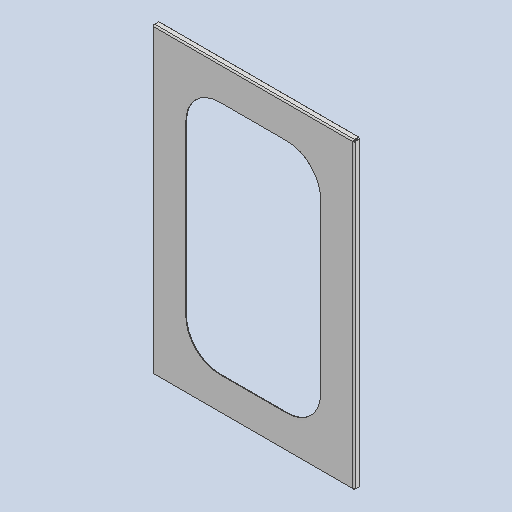
# Autodesk Inventor part: TapaCentral
Saved by Autodesk Inventor 2023 (Build 270158000, 158)
## iProperties
Created: 2022-11-27
Part Number: TapaCentral
Material: Generic
Document SubType Name: Sheet Metal
Designer: David
Density: 1 g/cm^3
Sheet Metal Rule: Default
Appearance: Default
Flat Pattern Width: 138.94 cm
Flat Pattern Length: 93.9405 cm
Flat Pattern Area: 13052.1 cm^2
Sheet Metal Width: 1389,405 mm
Sheet Metal Length: 939,405 mm
Sheet Metal Area: 1305213,601 mm^2
Author: David
Autodesk Inventor part; units mm, degrees
note: some values were not read from the file. Chosen so that the rebuilt part matches the saved one: corner form of "Plate4".
ref_plane "YZ Plane" through (0, 0, 0) normal (1, 0, 0) x (0, 1, 0)
ref_plane "XZ Plane" through (0, 0, 0) normal (0, 1, 0) x (-1, 0, 0)
ref_plane "XY Plane" through (0, 0, 0) normal (0, 0, 1) x (1, 0, 0)
sketch "Sketch1" plane through (0, 0, 0) normal (0, 0, 1) x (1, 0, 0)
  line L0 (-450, -675) -> (450, -675)
  line L1 (450, -675) -> (450, 675)
  line L2 (450, 675) -> (-450, 675)
  line L3 (-450, 675) -> (-450, -675)
  line L4 (-450, -675) -> (450, 675) construction
  line L5 (450, -675) -> (-450, 675) construction
  line L6 (-150, 525) -> (150, 525)
  line L7 (300, 375) -> (300, -375)
  line L8 (150, -525) -> (-150, -525)
  line L9 (-300, -375) -> (-300, 375)
  arc A0 (300, 375) -> (150, 525) centre (150, 375) ccw
  arc A1 (-150, 525) -> (-300, 375) centre (-150, 375) ccw
  arc A2 (-300, -375) -> (-150, -525) centre (-150, -375) ccw
  arc A3 (150, -525) -> (300, -375) centre (150, -375) ccw
  point P0 (0, 0)
  dimension "d0" = 900
  dimension "d1" = 1350
  dimension "d13" = 150
  dimension "d14" = 150
  dimension "d15" = 150
  dimension "d16" = 150
  dimension "d17" = 150
  measures "d0" distance of L2.end L1.end
  measures "d1" distance of L1.end L0.end
  measures "d13" distance between parallel lines of L2 L6
  measures "d14" radius of A0
  measures "d15" radius of A1
  measures "d16" radius of A2
  measures "d17" radius of A3
extrude "Plate3" add sketch "Sketch1" along normal blind 3.048
sketch "Sketch3" plane through (450, 671.952, 3.048) normal (0, 1, 0) x (-1, 0, 0)
  line L0 (900, 0) -> (0, 0)
  line L1 (0, 0) -> (0, -25)
  line L2 (0, -25) -> (900, -25)
  line L3 (900, -25) -> (900, 0)
  constraints: 6 end point, 1 horizontal, 1 perpendicular, 1 vertical
edge flange "Flange2" height 25 angle 90 thickness 3.048 bend radius 3.048 thickness toward (0, 1, 0) relief tear relief width 3.048 relief depth 1.524 corner gap 3.048 corner form 2 edges at (0, 675, 0) (-450, 0, 0) (450, 0, 0) (0, -675, 0) wall of the first edge with corners at (-450, 671.952, 3.048) (450, 671.952, 3.048) (450, 671.952, -21.952) (-450, 671.952, -21.952)
bend "Bend2"
corner "Corner2"
equation "\"d18\" = Thickness"
equation "\"d19\" = BendReliefWidth"
equation "\"d20\" = BendReliefDepth"
equation "\"d21\" = MinimumRemnant"
equation "\"d22\" = TransitionRadius"
equation "\"d25\" = BendRadius"
equation "\"d26\" = CornerReliefSize"
equation "\"d27\" = GapSize"
equation "\"d28\" = JacobiRadiusSize"
equation "\"BendRadius\" = Thickness"
equation "\"BendReliefWidth\" = Thickness"
equation "\"BendReliefDepth\" = 0.5 * Thickness"
equation "\"CornerReliefSize\" = 4 * Thickness"
equation "\"MinimumRemnant\" = 2 * Thickness"
equation "\"TransitionRadius\" = BendRadius"
equation "\"JacobiRadiusSize\" = BendRadius"
equation "\"GapSize\" = Thickness"
equation "\"Space5\" = 0"
equation "\"Space6\" = 0"
equation "\"Space7\" = 0"
equation "\"Thickness\" = 3.048"
body "Solid2"
